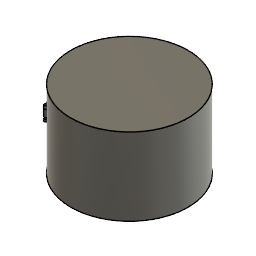
Ankita Water Bottle (Autodesk Fusion 360 archive; units mm, degrees)
design "dhakan"
part number: 2026-06-02-15-57-06-729
Autodesk Fusion 360 part; units mm, degrees
sketch "Sketch1" plane through (0, 0, 0) normal (0, 0, 1) x (1, 0, 0)
  line L0 (-11, 13) -> (-11, -48)
  line L1 (-11, 3) -> (-47.6999, 3)
  line L2 (-47.6999, 3) -> (-47.6999, -47)
  line L3 (-11, 8) -> (-52.6999, 8)
  line L4 (-52.6999, 8) -> (-52.6999, -47)
  line L5 (-11, 8) -> (30.6999, 8)
  line L6 (-11, 3) -> (25.6999, 3)
  line L7 (25.6999, 3) -> (25.6999, -47)
  line L8 (30.6999, 8) -> (30.6999, -47)
  line L9 (-52.6999, -47) -> (-47.6999, -47)
  line L10 (25.6999, -47) -> (30.6999, -47)
  dimension "d1" = 36.6999
  dimension "d2" = 50
  dimension "d3" = 5
  constraint vertical L0
  constraint coincident L0 L1.start
  constraint perpendicular L0 L1
  constraint perpendicular L1 L2
  constraint symmetric L0 L1.start L6.start
  constraint symmetric L0 L1.end L6.end
  constraint symmetric L0 L2.end L7.end
  constraint symmetric L0 L3.start L5.start
  constraint symmetric L0 L3.end L5.end
  constraint symmetric L0 L4.end L8.end
  constraint perpendicular L2 L9
  measures "d1" distance of L1.start L1.end
  measures "d2" distance of L1.end L2.end
revolve "Revolve1" add sketch "Sketch1" angle 360 about axis through (-11, 13, 0) along (0, -1, 0) contours L0 L1 L2 L3 L4 L9
thread "Thread1" "ISO Metric profile 72.0 M72x4 M72x4 6H" major diameter 72.4462 minor diameter 67.9699 pitch 4 angle 60 resizes the face on face at (-47.6543, -13.6667, 1.8293) from (-11, -40, 0) to (-11, -4, 0)
ref_plane "WorkPlane1" through (-52.6999, -17.6054, 0) normal (-1, 0, 0) x (0, 0, -1)
sketch "Sketch2" plane through (-52.6999, 0, 0) normal (-1, 0, 0) x (0, 0, 1)
  line L0 (-27.886, -34.3595) -> (31.8697, -34.3595) construction
  line L1 (31.8697, -34.3595) -> (31.8697, -9.7933) construction
  line L2 (31.8697, -9.7933) -> (-27.886, -9.7933) construction
  line L3 (-27.886, -9.7933) -> (-27.886, -34.3595) construction
  dimension "d8" = 10
  text T0 "Damnnn!" font "Arial" height 10 align left top in box 59.7557 x 24.5662 at (-27.886, -34.3595) x (1, 0) y (0, 1) spacing 1 kerned
emboss "Emboss1" depth 2 profiles "Sketch2" section 1 text T0 onto face at (-52.6481, -10.3333, 2.0786)
move_body "Move1" bodies 1 to x (1, 0, 0) y (0, 1, 0) z (0, 0, 1) at (0, -40, 0)
move_body "Move2" bodies 1 to x (1, 0, 0) y (0, 1, 0) z (0, 0, 1) at (0, -40, 0)
equation "d9 = 'Damnnn!'"
